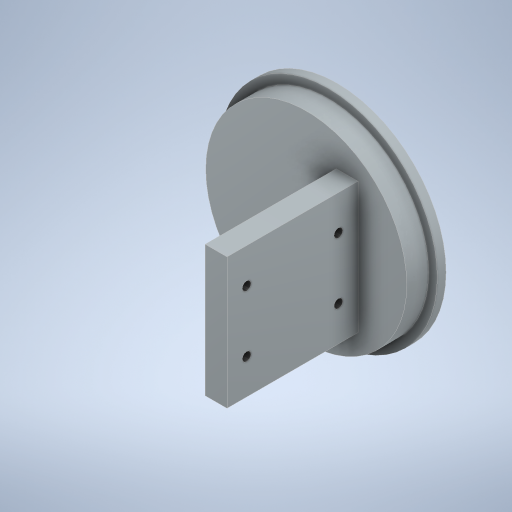
# Autodesk Inventor part: camera_poprywka
Saved by Autodesk Inventor 2024 (Build 280153000, 153)
## iProperties
Created: 2025-05-20
Part Number: camera_poprywka
Material: Tworzywo sztuczne PET
Document SubType Name: Modeling
Designer: Paweł
Density: 1.541 g/cm^3
Appearance: Ciemnoszara
Mass: 18.8565 g
Surface Area: 49.6372 cm^2
Volume: 12.2365 cm^3
Author: Paweł
Autodesk Inventor part; units mm, degrees
ref_plane "YZ Plane" through (0, 0, 0) normal (1, 0, 0) x (0, 1, 0)
ref_plane "XZ Plane" through (0, 0, 0) normal (0, 1, 0) x (-1, 0, 0)
ref_plane "XY Plane" through (0, 0, 0) normal (0, 0, 1) x (1, 0, 0)
sketch "Szkic1" plane through (0, 0, 0) normal (0, 0, 1) x (1, 0, 0)
  circle A0 centre (0, 0) radius 25
  dimension "d0" = 50
  constraints: 1 centre point, 1 coincident
  measures "d0" diameter of A0
extrude "Wyciągnięcie proste1" add sketch "Szkic1" along normal blind 2
sketch "Szkic2" plane through (0, 0, 2) normal (0, 0, 1) x (1, 0, 0)
  circle A0 centre (0, 0) radius 23
  dimension "d3" = 46
  constraints: 1 centre point, 1 coincident
  measures "d3" diameter of A0
extrude "Wyciągnięcie proste2" add sketch "Szkic2" along normal blind 5
sketch "Szkic3" plane through (0, 0, 7) normal (0, 0, 1) x (1, 0, 0)
  line L0 (6.8662, 15) -> (11.8662, 15)
  line L1 (11.8662, 15) -> (11.8662, -15)
  line L2 (11.8662, -15) -> (6.8662, -15)
  line L3 (6.8662, -15) -> (6.8662, 15)
  point P0 (0, 0)
  point P1 (6.8662, 0)
  dimension "d6" = 30
  dimension "d7" = 5
  constraints: 8 end point, 2 parallel, 1 horizontal, 1 horizontal alignment, 1 midpoint, 1 perpendicular
  measures "d6" distance of L2.end L0.start
  measures "d7" distance of L0.start L0.end
extrude "Wyciągnięcie proste3" add sketch "Szkic3" along normal blind 30
sketch "Szkic4" plane through (6.8662, -15, 7) normal (-1, 0, 0) x (0, 0, 1)
  circle A0 centre (4.5, 22) radius 1
  circle A1 centre (25.5, 22) radius 1
  circle A2 centre (4.5, 8) radius 1
  circle A3 centre (25.5, 8) radius 1
  line L0 (4.5, 22) -> (25.5, 22)
  line L1 (4.5, 22) -> (4.5, 8)
  line L2 (0, 30) -> (30, 30) projected
  line L3 (30, 30) -> (30, 0) projected
  point P0 (-7, 15)
  point P1 (15, 22)
  point P2 (15, 30)
  point P3 (4.5, 15)
  point P4 (30, 15)
  dimension "d10" = 2
  dimension "d11" = 2
  dimension "d12" = 2
  dimension "d13" = 2
  dimension "d14" = 14
  dimension "d15" = 21
  constraints: 4 centre point, 4 end point, 4 midpoint, 3 horizontal alignment, 3 vertical alignment, 1 horizontal, 1 vertical
  measures "d10" diameter of A0
  measures "d11" diameter of A1
  measures "d12" diameter of A2
  measures "d13" diameter of A3
  measures "d14" distance of L1.end L0.start
  measures "d15" distance of L0.end L0.start
extrude "Wyciągnięcie proste4" cut sketch "Szkic4" against normal blind 50
